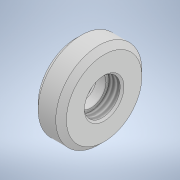
# Autodesk Inventor part: 711135
Saved by Autodesk Inventor 2022 (Build 260153000, 153)
## iProperties
Created: 2021-10-22
Part Number: 711135
Material: Типовые
Document SubType Name: Modeling
Designer: RaNSiD
Density: 1 g/cm^3
Appearance: По умолчанию
Author: RaNSiD
Autodesk Inventor part; units mm, degrees
ref_plane "YZ Plane" through (0, 0, 0) normal (1, 0, 0) x (0, 1, 0)
ref_plane "XZ Plane" through (0, 0, 0) normal (0, 1, 0) x (-1, 0, 0)
ref_plane "XY Plane" through (0, 0, 0) normal (0, 0, 1) x (1, 0, 0)
sketch "Эскиз1" plane through (0, 0, 0) normal (0, 0, 1) x (1, 0, 0)
  line L0 (0, 0) -> (0, 20)
  line L1 (0, 20) -> (2.8284, 22.8284)
  line L2 (0, 0) -> (15, 0)
  line L3 (15, 0) -> (15, 20)
  line L4 (15, 20) -> (12.1716, 22.8284)
  line L5 (2.8284, 22.8284) -> (12.1716, 22.8284)
  dimension "d0" = 20
  dimension "d1" = 4
  dimension "d2" = 135
  dimension "d3" = 15
  dimension "d4" = 4
  dimension "d5" = 135
  constraints: 12 end point, 2 horizontal, 1 perpendicular, 1 vertical
  measures "d0" distance of L0.start L0.end
  measures "d1" distance of L0.end L1.end
  measures "d2" angle of L0 L1
  measures "d3" distance of L0.start L2.end
  measures "d4" distance of L3.end L4.end
  measures "d5" angle of L4 L3
revolve "Вращение1" add sketch "Эскиз1" angle 360 about axis through (0, 0, 0) along (1, 0, 0)
sketch "Эскиз2" plane through (0, 0, 0) normal (-1, 0, 0) x (0, 0, 1)
  point P0 (0, 0)
  point P1 (0, 18)
  point P2 (-15.5885, 9)
  point P3 (-15.5885, -9)
  point P4 (0, -18)
  point P5 (15.5885, -9)
  point P6 (15.5885, 9)
  dimension "d7" = 18
  dimension "d10" = 360
  constraints: 1 vertical alignment, 7 other
  measures "d7" distance of point (0, 0) point (0, 18)
hole "Отверстие1" at (0, 18, 0) at (0, 9, -15.5885) at (0, -9, -15.5885) at (0, -18, 0) at (0, -9, 15.5885) at (0, 9, 15.5885) direction (1, 0, 0) diameter 4 depth 4
sketch "Эскиз3" plane through (0, 0, 0) normal (0, 0, 1) x (1, 0, 0)
  line L0 (0, 0) -> (0, 11)
  line L1 (0, 11) -> (3, 8)
  line L2 (3, 8) -> (8, 8)
  line L3 (8, 8) -> (8, 9.5)
  line L4 (8, 9.5) -> (14, 9.5)
  line L5 (14, 9.5) -> (15, 10.5)
  line L6 (15, 10.5) -> (15, 0)
  line L7 (15, -20) -> (15, 20) projected
  line L8 (0, 0) -> (15, 0)
  dimension "d19" = 45
  dimension "d21" = 45
  dimension "d22" = 16
  dimension "d23" = 19
  dimension "d24" = 5
  dimension "d26" = 10.5
  dimension "d30" = 6
  constraints: 16 end point, 3 perpendicular, 2 vertical, 1 midpoint
  measures "d19" angle of L6 L5
  measures "d21" angle of L0 L1
  measures "d22" diameter of L2 L8
  measures "d23" diameter of L4 L8
  measures "d24" distance of L1.end L2.end
  measures "d26" distance of L5.end L6.end
  measures "d30" distance of L3.end L4.end
revolve "Вращение2" cut sketch "Эскиз3" angle 360 about axis through (0, 0, 0) along (1, 0, 0)
thread "Резьба1" size "M20x2.5" class "6H" standard "ANSI Metric M Profile" full length
